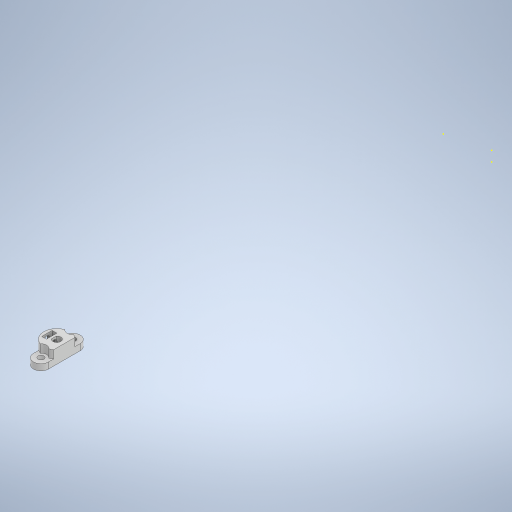
# Autodesk Inventor part: Acople3
Saved by Autodesk Inventor 2024 (Build 280153000, 153)
## iProperties
Created: 2024-08-27
Part Number: Acople3
Material: Generic
Document SubType Name: Modeling
Designer: drica
Density: 1 g/cm^3
Appearance: Default
Author: drica
Autodesk Inventor part; units mm, degrees
ref_plane "YZ Plane" through (0, 0, 0) normal (1, 0, 0) x (0, 1, 0)
ref_plane "XZ Plane" through (0, 0, 0) normal (0, 1, 0) x (-1, 0, 0)
ref_plane "XY Plane" through (0, 0, 0) normal (0, 0, 1) x (1, 0, 0)
sketch "Sketch1" plane through (0, 0, 0) normal (0, 1, 0) x (-1, 0, 0)
  line L0 (31.678, 204.1316) -> (31.678, 201.3316)
  line L1 (31.678, 201.3316) -> (31.678, 206.9316)
  circle A0 centre (28.8694, 204.1316) radius 2.1
  line L2 (26.7694, 204.1316) -> (30.3694, 204.1316)
  line L3 (30.3694, 204.1316) -> (30.3694, 202.6619)
  line L4 (30.3694, 202.6619) -> (30.3694, 205.6012)
  line L5 (30.3694, 204.1316) -> (31.678, 204.1316)
  line L6 (31.678, 201.3316) -> (34.178, 201.3316)
  line L7 (34.178, 201.3316) -> (34.178, 206.9316)
  line L8 (34.178, 206.9316) -> (31.678, 206.9316)
  line L9 (31.678, 206.9316) -> (31.678, 201.3316)
  circle A1 centre (28.8694, 204.1316) radius 8.5
  circle A2 centre (28.8694, 212.6316) radius 1.55
  circle A3 centre (28.8694, 195.6316) radius 1.55
  line L10 (22.8334, 207.9209) -> (34.9053, 207.9209)
  line L11 (34.9053, 207.9209) -> (34.9053, 200.3422)
  line L12 (34.9053, 200.3422) -> (22.8334, 200.3422)
  line L13 (22.8334, 200.3422) -> (22.8334, 207.9209)
  line L14 (22.8334, 207.9209) -> (34.9053, 200.3422) construction
  line L15 (34.9053, 207.9209) -> (22.8334, 200.3422) construction
  line L16 (22.8334, 200.3422) -> (25.8027, 200.3422)
  line L17 (25.8027, 200.3422) -> (25.8027, 207.9209)
  line L18 (25.8027, 207.9209) -> (22.8334, 207.9209)
  line L19 (22.8334, 207.9209) -> (22.8334, 200.3422)
  dimension "d1" = 2.8
  dimension "d2" = 5.6
  dimension "d3" = 4.2
  dimension "d5" = 2.5
  dimension "d6" = 17
  dimension "d7" = 3.1
  dimension "d8" = 3.1
  constraints: 40 end point, 6 parallel, 5 point on circle, 4 centre point, 4 horizontal, 3 perpendicular, 3 point on line, 2 midpoint, 2 vertical, 1 coincident
  measures "d1" distance of L0.start L0.end
  measures "d2" distance of L0.end L1.end
  measures "d3" diameter of A0
  measures "d5" distance of L8.end L7.end
  measures "d6" diameter of A1
  measures "d7" diameter of A2
  measures "d8" diameter of A3
extrude "Extrusion1" add sketch "Sketch1" along normal blind 7 contours L10 L11 L12 L17
sketch "Sketch2" plane through (0, 0, 0) normal (0, -1, 0) x (1, 0, 0)
  point P0 (0, 0)
sketch "Sketch3" plane through (0, 0, 0) normal (0, -1, 0) x (1, 0, 0)
  circle A0 centre (-28.8694, 204.1316) radius 2.1 projected
  circle A1 centre (-28.8694, 204.1316) radius 8.5
  circle A2 centre (-28.8694, 212.6316) radius 1.55
  circle A3 centre (-28.8694, 195.6316) radius 1.55
  circle A4 centre (-28.8694, 212.6316) radius 3
  circle A5 centre (-28.8694, 195.6316) radius 3
  line L0 (-31.8694, 212.6316) -> (-31.8694, 195.6316)
  line L1 (-25.8694, 195.6316) -> (-25.8694, 212.6316)
  point P0 (0, 0)
  point P1 (-25.9164, 212.1021)
  point P2 (-31.8223, 212.1021)
  point P3 (-31.8694, 212.0845)
  point P4 (-31.8694, 196.1786)
  point P5 (-31.8223, 196.161)
  point P6 (-25.9164, 196.161)
  point P7 (-25.8694, 196.1786)
  point P8 (-25.8694, 212.0845)
  dimension "d11" = 17
  dimension "d12" = 3.1
  dimension "d13" = 3.1
  dimension "d14" = 6
  dimension "d15" = 6
  constraints: 6 point on circle, 5 centre point, 4 end point, 3 coincident, 3 tangent
  measures "d11" diameter of A1
  measures "d12" diameter of A2
  measures "d13" diameter of A3
  measures "d14" diameter of A4
  measures "d15" diameter of A5
extrude "Extrusion4" add sketch "Sketch3" along normal blind 2.3 contours L1 A1 A5 L0 A4 | A1 A4 L1 | L1 A5 A1 | A4 A1 A2 | A1 A2 A4 | A5 A1 A3 | A1 A3 A5 | A1 L0 A4 | A5 L0 A1
sketch "Sketch5" plane through (0, 0, 0) normal (0, -1, 0) x (1, 0, 0)
  line L0 (-34.9053, 207.9209) -> (-25.8027, 207.9209) projected
  line L1 (-31.8694, 200.3422) -> (-31.8694, 201.3316) projected
  line L2 (-34.9053, 207.9209) -> (-31.8694, 207.9209)
  line L3 (-31.8694, 207.9209) -> (-31.8694, 200.3422)
  line L4 (-31.8694, 200.3422) -> (-34.9053, 200.3422)
  line L5 (-34.9053, 200.3422) -> (-34.9053, 207.9209)
  line L6 (-34.178, 201.3316) -> (-31.678, 201.3316) projected
  line L7 (-31.678, 206.9316) -> (-34.178, 206.9316) projected
  line L8 (-34.178, 201.3316) -> (-31.8694, 201.3316)
  line L9 (-31.8694, 201.3316) -> (-31.8694, 206.9316)
  line L10 (-31.8694, 206.9316) -> (-34.178, 206.9316)
  line L11 (-34.178, 206.9316) -> (-34.178, 201.3316)
  point P0 (0, 0)
  constraints: 16 end point, 4 parallel, 2 horizontal, 2 perpendicular, 2 point on line
extrude "Extrusion5" add sketch "Sketch5" along normal blind 2.3 contours L0 L3 L7 L11 L6 L1 L4 L5
sketch "Sketch6" plane through (-25.8694, 0, 200.3422) normal (1, 0, 0) x (0, 0, -1)
  line L0 (-9.2808, 8.2816) -> (1.9224, 8.2816)
  line L1 (1.9224, 8.2816) -> (1.9224, -4.0318)
  line L2 (1.9224, -4.0318) -> (-9.2808, -4.0318)
  line L3 (-9.2808, -4.0318) -> (-9.2808, 8.2816)
  point P0 (200.3422, 0)
  constraints: 8 end point, 2 parallel, 1 horizontal, 1 perpendicular
extrude "Extrusion6" cut sketch "Sketch6" along normal blind 2.3
sketch "Sketch7" plane through (-25.8694, 0, 212.6316) normal (1, 0, 0) x (0, 0, -1)
  point P0 (212.6316, 0)
sketch "Sketch8" plane through (0, 7, 0) normal (0, 1, 0) x (1, 0, 0)
  line L0 (-31.678, -201.3316) -> (-31.678, -206.9316) projected
  line L1 (-31.678, -206.9316) -> (-34.178, -206.9316) projected
  line L2 (-34.178, -206.9316) -> (-34.178, -201.3316) projected
  line L3 (-34.178, -201.3316) -> (-31.678, -201.3316) projected
  circle A0 centre (-28.8694, -204.1316) radius 2.1 projected
  line L4 (-25.8694, -207.9209) -> (-25.8694, -200.3422) projected
  line L5 (-25.8694, -200.3422) -> (-34.9053, -200.3422) projected
  line L6 (-34.9053, -200.3422) -> (-34.9053, -207.9209) projected
  line L7 (-34.9053, -207.9209) -> (-25.8694, -207.9209) projected
  point P0 (0, 0)
extrude "Extrusion7" cut sketch "Sketch8" against normal blind 1.7
sketch "Sketch9" plane through (0, 5.3, 0) normal (0, 1, 0) x (1, 0, 0)
  line L0 (-31.678, -201.3316) -> (-31.678, -206.9316) projected
  line L1 (-34.178, -206.9316) -> (-31.8694, -206.9316) projected
  line L2 (-31.678, -201.3316) -> (-34.178, -201.3316)
  line L3 (-34.178, -201.3316) -> (-34.178, -206.9316)
  line L4 (-34.178, -206.9316) -> (-31.678, -206.9316)
  line L5 (-31.678, -206.9316) -> (-31.678, -201.3316)
  point P0 (0, 0)
  constraints: 8 end point, 2 parallel, 1 horizontal, 1 perpendicular
extrude "Extrusion8" cut sketch "Sketch9" against normal through all
sketch "Sketch10" plane through (-34.9053, -2.3, 200.3422) normal (-1, 0, 0) x (0, 0, 1)
  line L0 (6.5893, 7.6) -> (0.9893, 7.6) projected
  line L1 (3.7893, 7.6) -> (3.7893, 0)
  line L2 (5.8893, 0) -> (1.6893, 0) projected
  line L3 (3.7893, 2.0731) -> (3.7893, 5.5269) construction
  line L4 (3.7893, 3.8) -> (3.7893, 2.7114)
  line L5 (3.7893, 4.8886) -> (3.7893, 2.7114) construction
  line L6 (2.1893, 4.8886) -> (2.1893, 2.7114)
  line L7 (5.3893, 2.7114) -> (5.3893, 4.8886)
  arc A0 (5.3893, 4.8886) -> (2.1893, 4.8886) centre (3.7893, 4.8886) ccw
  arc A1 (2.1893, 2.7114) -> (5.3893, 2.7114) centre (3.7893, 2.7114) ccw
  point P0 (-200.3422, 2.3)
  dimension "d39" = 3.2
  constraints: 16 end point, 5 midpoint, 4 point on circle, 4 tangent, 2 centre point, 2 point on line, 1 collinear, 1 parallel
  measures "d39" diameter of A1
fillet "Fillet1" radius 0.7 2 edges at (-34.9053, 1.5, 207.9209) (-34.9053, 1.5, 200.3422)
fillet "Fillet2" radius 1 2 edges at (-25.8694, 2.65, 207.9209) (-25.8694, 2.65, 200.3422)
sketch "Sketch11" plane through (0, 5.3, 0) normal (0, 1, 0) x (1, 0, 0)
  circle A0 centre (-28.8694, -204.1316) radius 2.1 projected
  circle A1 centre (-28.8694, -204.1316) radius 2.1
  line L0 (-26.7694, -204.1316) -> (-30.4694, -204.1316)
  line L1 (-30.4694, -204.1316) -> (-30.4694, -202.7714)
  line L2 (-30.4694, -202.7714) -> (-30.4694, -205.4917)
  point P0 (0, 0)
  dimension "d36" = 3.7
  constraints: 6 end point, 3 point on circle, 1 centre point, 1 coincident, 1 horizontal, 1 perpendicular, 1 point on line
  measures "d36" distance of L0.start L0.end
extrude "Extrusion10" add sketch "Sketch11" against normal up to surface (7.6 mm away) contours L1 L2 A0
extrude "Extrusion11" cut sketch "Sketch10" against normal blind 6
sketch "Sketch12" plane through (0, 5.3, 0) normal (0, 1, 0) x (1, 0, 0)
  circle A0 centre (-28.8694, -212.6316) radius 1.55 projected
  circle A1 centre (-28.8694, -212.6316) radius 3
  circle A2 centre (-28.8694, -195.6316) radius 1.55 projected
  circle A3 centre (-28.8694, -195.6316) radius 3
  arc A4 (-30.4694, -205.4917) -> (-30.4694, -202.7714) centre (-28.8694, -204.1316) ccw projected
  circle A5 centre (-28.8694, -204.1316) radius 6.9874
  arc A6 (-25.8694, -201.3422) -> (-26.8694, -200.3422) centre (-26.8694, -201.3422) ccw projected
  line L0 (-34.2053, -200.3422) -> (-26.8694, -200.3422) projected
  arc A7 (-34.2053, -200.3422) -> (-34.9053, -201.0422) centre (-34.2053, -201.0422) ccw projected
  line L1 (-34.9053, -207.2209) -> (-34.9053, -201.0422) projected
  arc A8 (-34.9053, -207.2209) -> (-34.2053, -207.9209) centre (-34.2053, -207.2209) ccw projected
  line L2 (-26.8694, -207.9209) -> (-34.2053, -207.9209) projected
  arc A9 (-26.8694, -207.9209) -> (-25.8694, -206.9209) centre (-26.8694, -206.9209) ccw projected
  line L3 (-25.8694, -201.3422) -> (-25.8694, -206.9209) projected
  line L4 (-31.678, -206.9316) -> (-31.678, -201.3316) projected
  line L5 (-34.178, -206.9316) -> (-31.678, -206.9316) projected
  line L6 (-34.178, -201.3316) -> (-34.178, -206.9316) projected
  line L7 (-31.678, -201.3316) -> (-34.178, -201.3316) projected
  arc A10 (-30.4694, -205.4917) -> (-30.4694, -202.7714) centre (-28.8694, -204.1316) ccw projected
  line L8 (-30.4694, -205.4917) -> (-30.4694, -202.7714) projected
  point P0 (0, 0)
  point P1 (-31.1849, -197.539)
  point P2 (-31.1849, -210.7242)
  point P3 (-26.5538, -210.7242)
  point P4 (-26.5538, -197.539)
  dimension "d42" = 6
  dimension "d43" = 6
  constraints: 3 centre point, 3 coincident
  measures "d42" diameter of A1
  measures "d43" diameter of A3
extrude "Extrusion12" add sketch "Sketch12" against normal up to surface (7.6 mm away) contours A1 A5 A3
sketch "Sketch13" plane through (0, 0, 0) normal (0, 1, 0) x (1, 0, 0)
  circle A0 centre (-28.8694, -212.6316) radius 1.55 projected
  circle A1 centre (-28.8694, -212.6316) radius 4
  circle A2 centre (-28.8694, -195.6316) radius 1.55 projected
  circle A3 centre (-28.8694, -195.6316) radius 4
  line L0 (-32.8694, -212.6316) -> (-32.8694, -195.6316)
  line L1 (-24.8694, -212.6316) -> (-24.8694, -195.6316)
  line L2 (-31.678, -201.3316) -> (-34.178, -201.3316) projected
  line L3 (-34.178, -206.9316) -> (-31.678, -206.9316) projected
  line L4 (-31.678, -201.3316) -> (-32.928, -201.3316)
  line L5 (-32.928, -201.3316) -> (-32.928, -206.9316)
  line L6 (-32.928, -206.9316) -> (-31.678, -206.9316)
  line L7 (-31.678, -206.9316) -> (-31.678, -201.3316)
  point P0 (0, 0)
  point P1 (-32.8694, -201.3316)
  point P2 (-32.8694, -206.9316)
  dimension "d46" = 8
  dimension "d47" = 8
  constraints: 12 end point, 4 point on circle, 2 centre point, 2 coincident, 2 parallel, 2 tangent, 1 horizontal, 1 midpoint, 1 perpendicular
  measures "d46" diameter of A1
  measures "d47" diameter of A3
extrude "Extrusion13" add sketch "Sketch13" against normal up to surface (2.3 mm away) contours A1 | A1 L0 L3 L7 L2 A3 L1 | A3
sketch "Sketch14" plane through (0, 5.3, 0) normal (0, 1, 0) x (1, 0, 0)
  line L0 (-24.8694, -212.6316) -> (-24.8694, -209.8608) projected
  line L1 (-24.8694, -198.4023) -> (-24.8694, -195.6316) projected
  line L2 (-24.8694, -209.8608) -> (-24.8694, -198.4023)
  line L3 (-24.8694, -198.4023) -> (-21.4183, -198.4023)
  line L4 (-21.4183, -198.4023) -> (-21.2342, -210.9453)
  line L5 (-21.2342, -210.9453) -> (-24.8694, -209.8608)
  point P0 (0, 0)
  constraints: 8 end point, 1 collinear, 1 perpendicular
extrude "Extrusion14" cut sketch "Sketch14" against normal through all
sketch "Sketch16" plane through (-34.9053, 0.4114, 202.5316) normal (1, 0, 0) x (0, 0, -1)
  line L0 (0, 0) -> (0, 2.1771) projected
  arc A0 (0, 2.1771) -> (-3.2, 2.1771) centre (-1.6, 2.1771) ccw projected
  line L1 (-3.2, 2.1771) -> (-3.2, 0) projected
  arc A1 (-3.2, 0) -> (0, 0) centre (-1.6, 0) ccw projected
  point P0 (202.5316, -0.4114)
extrude "Extrusion16" cut sketch "Sketch16" against normal blind 10
sketch "Sketch17" plane through (0, 0, 0) normal (0, 1, 0) x (1, 0, 0)
  arc A0 (-32.8694, -209.8608) -> (-31.1849, -210.7242) centre (-28.8694, -204.1316) ccw projected
  line L0 (-32.8694, -209.8608) -> (-32.8694, -212.6316) projected
  arc A1 (-32.8694, -212.6316) -> (-24.8694, -212.6316) centre (-28.8694, -212.6316) ccw projected
  line L1 (-24.8694, -212.6316) -> (-24.8694, -209.8608) projected
  arc A2 (-26.5538, -210.7242) -> (-24.8694, -209.8608) centre (-28.8694, -204.1316) ccw projected
  arc A3 (-26.5538, -210.7242) -> (-31.1849, -210.7242) centre (-28.8694, -212.6316) ccw projected
  circle A4 centre (-28.8694, -212.6316) radius 1.55 projected
  arc A5 (-31.1849, -197.539) -> (-32.8694, -198.4023) centre (-28.8694, -204.1316) ccw projected
  arc A6 (-31.1849, -197.539) -> (-26.5538, -197.539) centre (-28.8694, -195.6316) ccw projected
  arc A7 (-24.8694, -198.4023) -> (-26.5538, -197.539) centre (-28.8694, -204.1316) ccw projected
  line L2 (-24.8694, -198.4023) -> (-24.8694, -195.6316) projected
  arc A8 (-24.8694, -195.6316) -> (-32.8694, -195.6316) centre (-28.8694, -195.6316) ccw projected
  line L3 (-32.8694, -195.6316) -> (-32.8694, -198.4023) projected
  circle A9 centre (-28.8694, -195.6316) radius 1.55 projected
  point P0 (0, 0)
extrude "Extrusion17" add sketch "Sketch17" along normal blind 1
sketch "Sketch18" plane through (0, 0, 0) normal (0, 1, 0) x (1, 0, 0)
  line L0 (-30.2904, -205.6777) -> (-31.678, -205.6777) projected
  arc A0 (-30.2904, -205.6777) -> (-30.2904, -202.5854) centre (-28.8694, -204.1316) ccw projected
  line L1 (-31.678, -202.5854) -> (-30.2904, -202.5854) projected
  line L2 (-31.678, -202.5854) -> (-31.678, -205.6777) projected
  point P0 (0, 0)
sketch "Sketch19" plane through (0, 5.3, 0) normal (0, 1, 0) x (1, 0, 0)
  line L0 (-30.4694, -205.4917) -> (-30.4694, -202.7714) projected
  arc A0 (-30.4694, -205.4917) -> (-30.4694, -202.7714) centre (-28.8694, -204.1316) ccw projected
  point P0 (0, 0)
extrude "Extrusion18" cut sketch "Sketch19" against normal through all
sketch "Sketch20" plane through (0, 5.3, 0) normal (0, 1, 0) x (1, 0, 0)
  point P0 (0, 0)
body "Solid1"
